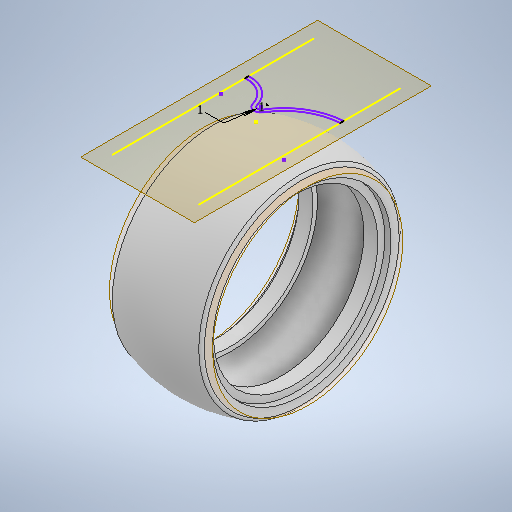
# Autodesk Inventor part: tire
Saved by Autodesk Inventor 2025 (Build 290162000, 162)
## iProperties
Created: 2024-04-11
Part Number: tire
Material: Generic
Document SubType Name: Modeling
Designer: bartek
Density: 1 g/cm^3
Appearance: Default
Author: bartek
Autodesk Inventor part; units mm, degrees
ref_plane "YZ Plane" through (0, 0, 0) normal (1, 0, 0) x (0, 1, 0)
ref_plane "XY Plane" through (0, 0, 0) normal (0, 0, 1) x (1, 0, 0)
sketch "Sketch1" plane through (0, 0, 0) normal (0, 0, 1) x (1, 0, 0)
  line L0 (-13.27, 0) -> (13.27, 0)
  line L1 (-7.43, 23.94) -> (-11.49, 23.94)
  line L2 (-11.49, 23.94) -> (-11.49, 25.97)
  line L3 (-11.49, 25.97) -> (-13.27, 25.97)
  line L4 (-13.27, 25.97) -> (-13.27, 28.3865)
  line L5 (0, 0) -> (0, 31.38)
  line L6 (7.43, 23.94) -> (11.49, 23.94)
  line L7 (11.49, 23.94) -> (11.49, 25.97)
  line L8 (11.49, 25.97) -> (13.27, 25.97)
  line L9 (13.27, 25.97) -> (13.27, 28.3865)
  arc A0 (12.5866, 29.335) -> (-12.5866, 29.335) centre (0, -8.3769) ccw
  arc A1 (-12.5866, 29.335) -> (-13.27, 28.3865) centre (-12.27, 28.3865) ccw
  arc A2 (13.27, 28.3865) -> (12.5866, 29.335) centre (12.27, 28.3865) ccw
  line L10 (-7.43, 25.266) -> (-10.164, 25.266)
  line L11 (-10.164, 25.266) -> (-10.164, 27.296)
  line L12 (-10.164, 27.296) -> (-11.944, 27.296)
  line L13 (-11.944, 27.296) -> (-11.944, 28.1508)
  arc A3 (11.944, 28.1508) -> (-11.944, 28.1508) centre (0, -8.3769) ccw
  line L14 (11.944, 28.1508) -> (11.944, 27.296)
  line L15 (11.944, 27.296) -> (10.164, 27.296)
  line L16 (10.164, 27.296) -> (10.164, 25.266)
  line L17 (10.164, 25.266) -> (7.43, 25.266)
  line L18 (-7.43, 25.266) -> (-7.43, 23.94)
  line L19 (7.43, 25.266) -> (7.43, 23.94)
  point P0 (-13.27, 29.1)
  point P1 (13.27, 29.1)
  dimension "d0" = 26.54
  dimension "d1" = 23.94
  dimension "d2" = 7.43
  dimension "d3" = 4.06
  dimension "d4" = 2.03
  dimension "d5" = 1.78
  dimension "d6" = 3.13
  dimension "d7" = 31.38
  dimension "d8" = 1
  dimension "d9" = 1
  dimension "d10" = 1.326
  constraints: 40 end point, 11 point on circle, 6 perpendicular, 5 symmetric about line, 4 centre point, 4 tangent, 2 horizontal, 2 midpoint, 2 point on line, 2 vertical, 1 parallel, 8 other
  measures "d0" distance of L0.start L0.end
  measures "d1" vertical distance of L5.start L1.start
  measures "d2" horizontal distance of L5.start L1.start
  measures "d3" distance of L1.start L1.end
  measures "d4" distance of L1.end L2.end
  measures "d5" distance of L2.end L3.end
  measures "d6" distance of L3.end point (-13.27, 29.1)
  measures "d7" distance of L5.start L5.end
  measures "d8" radius of A1
  measures "d9" radius of A2
  measures "d10" radial gap between concentric circles of A0 A3
revolve "Revolution1" add sketch "Sketch1" angle 360 about axis through (-13.27, 0, 0) along (1, 0, 0)
sketch "Sketch2" plane through (0, 0, 0) normal (0, 0, 1) x (1, 0, 0)
  arc A0 (12.5866, 29.335) -> (-12.5866, 29.335) centre (0, -8.3769) ccw projected
  arc A1 (14.9927, 27.6878) -> (-15.1313, 27.6298) centre (0, -8.3769) ccw
  line L0 (-21.1631, 0) -> (21.0186, 0) projected
  point P0 (0, 0)
  dimension "d12" = 0.7
  constraints: 2 point on circle, 1 centre point
  measures "d12" radial gap between concentric circles of A0 A1
surface revolve "RevolutionSrf1" sketch "Sketch2" angle 360 about axis through (-10, 0, 0) along (1, 0, 0) shown yes curves A1
ref_plane "Work Plane1" through (0, 36.5125, 0) normal (0, 1, 0) x (-1, 0, 0)
sketch "Sketch3" plane through (0, 36.5125, 0) normal (0, 1, 0) x (-1, 0, 0)
  line L0 (12.5866, 29.335) -> (12.5866, -29.335) projected
  line L1 (-12.5866, 29.335) -> (-12.5866, -29.335) projected
  arc A0 (-12.5866, -12.8966) -> (2.1673, -3.8903) centre (-13.8064, 5.6896) ccw
  arc A1 (3.9904, -4.1445) -> (12.5866, -10.3655) centre (12.1261, -1.9522) ccw
  arc A2 (3.9904, -4.1445) -> (2.1673, -3.8903) centre (3.0249, -4.4047) ccw
  arc A3 (-12.5866, -11.8943) -> (1.3097, -3.376) centre (-13.8064, 5.6896) ccw
  arc A4 (4.956, -3.8843) -> (1.3097, -3.376) centre (3.0249, -4.4047) ccw
  arc A5 (4.956, -3.8843) -> (12.5866, -9.3638) centre (12.1261, -1.9522) ccw
  line L2 (12.5866, -10.3655) -> (12.5866, -9.3638)
  line L3 (-12.5866, -12.8966) -> (-12.5866, -11.8943)
  point P0 (0, 0)
  dimension "d15" = 1
  dimension "d16" = 1
  constraints: 12 point on circle, 6 centre point, 4 end point, 4 point on line, 2 tangent, 1 other
  measures "d15" radius of A2
  measures "d16" radial gap between concentric circles of A2 A4
body "Solid1"
body "Srf1"
